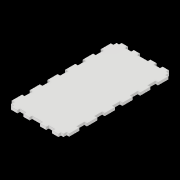
# Autodesk Inventor part: Bottom
Saved by Autodesk Inventor 2018 (Build 220112000, 112)
## iProperties
Created: 2018-03-12
Part Number: Bottom
Material: UHMW, White
Document SubType Name: Modeling
Designer: gaine
Density: 0.94 g/cm^3
Appearance: Smooth - White
Author: gaine
Autodesk Inventor part; units mm, degrees
ref_plane "YZ Plane" through (0, 0, 0) normal (1, 0, 0) x (0, 1, 0)
ref_plane "XZ Plane" through (0, 0, 0) normal (0, 1, 0) x (-1, 0, 0)
ref_plane "XY Plane" through (0, 0, 0) normal (0, 0, 1) x (1, 0, 0)
sketch "Sketch1" plane through (0, 0, 0) normal (0, 1, 0) x (-1, 0, 0)
  line L0 (36.5552, 136.6167) -> (36.5552, 130.2667)
  line L1 (21.3152, 130.2667) -> (21.3152, 136.6167)
  line L2 (58.1452, 96.9292) -> (64.4952, 96.9292)
  line L3 (64.4952, 77.8792) -> (58.1452, 77.8792)
  line L4 (58.1452, 52.4792) -> (64.4952, 52.4792)
  line L5 (64.4952, 33.4292) -> (58.1452, 33.4292)
  line L6 (58.1452, 8.0292) -> (64.4952, 8.0292)
  line L7 (64.4952, -1.4958) -> (-62.2762, -1.4958) construction
  line L8 (-7.1455, 136.6167) -> (-7.1455, -139.6083) construction
  line L9 (58.1452, 96.9292) -> (58.1452, 77.8792)
  line L10 (58.1452, 33.4292) -> (58.1452, 52.4792)
  line L11 (36.5552, 130.2667) -> (21.3152, 130.2667)
  line L12 (-50.8462, 136.6167) -> (-50.8462, 130.2667)
  line L13 (-20.3662, 136.6167) -> (-20.3662, 130.2667)
  line L14 (-35.6062, 130.2667) -> (-35.6062, 136.6167)
  line L15 (-78.7862, 122.3292) -> (-72.4362, 122.3292)
  line L16 (-72.4362, 96.9292) -> (-78.7862, 96.9292)
  line L17 (-78.7862, 77.8792) -> (-72.4362, 77.8792)
  line L18 (-72.4362, 52.4792) -> (-78.7862, 52.4792)
  line L19 (-78.7862, 33.4292) -> (-72.4362, 33.4292)
  line L20 (-72.4362, 8.0292) -> (-78.7862, 8.0292)
  line L21 (-72.4362, 96.9292) -> (-72.4362, 77.8792)
  line L22 (-72.4362, 33.4292) -> (-72.4362, 52.4792)
  line L23 (-50.8462, 130.2667) -> (-35.6062, 130.2667)
  line L24 (36.5552, -139.6083) -> (36.5552, -133.2583)
  line L25 (6.0752, -139.6083) -> (6.0752, -133.2583)
  line L26 (21.3152, -133.2583) -> (21.3152, -139.6083)
  line L27 (64.4952, -125.3208) -> (58.1452, -125.3208)
  line L28 (58.1452, -99.9208) -> (64.4952, -99.9208)
  line L29 (64.4952, -80.8708) -> (58.1452, -80.8708)
  line L30 (58.1452, -55.4708) -> (64.4952, -55.4708)
  line L31 (64.4952, -36.4208) -> (58.1452, -36.4208)
  line L32 (58.1452, -11.0208) -> (64.4952, -11.0208)
  line L33 (-7.1455, -139.6083) -> (-7.1455, 136.6167) construction
  line L34 (58.1452, -99.9208) -> (58.1452, -80.8708)
  line L35 (58.1452, -36.4208) -> (58.1452, -55.4708)
  line L36 (36.5552, -133.2583) -> (21.3152, -133.2583)
  line L37 (-72.4362, -55.4708) -> (-78.7862, -55.4708)
  line L38 (-78.7862, -80.8708) -> (-72.4362, -80.8708)
  line L39 (-72.4362, -99.9208) -> (-72.4362, -80.8708)
  line L40 (-50.8462, -139.6083) -> (-50.8462, -133.2583)
  line L41 (-20.3662, -139.6083) -> (-20.3662, -133.2583)
  line L42 (-35.6062, -133.2583) -> (-35.6062, -139.6083)
  line L43 (-72.4362, -99.9208) -> (-78.7862, -99.9208)
  line L44 (-78.7862, -125.3208) -> (-72.4362, -125.3208)
  line L45 (-50.8462, -133.2583) -> (-35.6062, -133.2583)
  line L46 (-72.4362, -36.4208) -> (-72.4362, -55.4708)
  line L47 (-78.7862, -36.4208) -> (-72.4362, -36.4208)
  line L48 (-72.4362, -11.0208) -> (-78.7862, -11.0208)
  line L49 (51.7952, 136.6167) -> (36.5552, 136.6167)
  line L50 (-20.3662, 136.6167) -> (-35.6062, 136.6167)
  line L51 (-50.8462, 136.6167) -> (-66.0862, 136.6167)
  line L52 (64.4952, 96.9292) -> (64.4952, 122.3292)
  line L53 (64.4952, 52.4792) -> (64.4952, 77.8792)
  line L54 (58.1452, 8.0292) -> (58.1452, -11.0208)
  line L55 (64.4952, 8.0292) -> (64.4952, 33.4292)
  line L56 (64.4952, -36.4208) -> (64.4952, -11.0208)
  line L57 (64.4952, -80.8708) -> (64.4952, -55.4708)
  line L58 (58.1452, -125.3208) -> (58.1452, -133.2583)
  line L59 (-72.4362, -133.2583) -> (-72.4362, -125.3208)
  line L60 (-72.4362, 8.0292) -> (-72.4362, -11.0208)
  line L61 (-72.4362, 122.3292) -> (-72.4362, 130.2667)
  line L62 (-78.7862, 122.3292) -> (-78.7862, 96.9292)
  line L63 (-78.7862, 77.8792) -> (-78.7862, 52.4792)
  line L64 (-78.7862, 33.4292) -> (-78.7862, 8.0292)
  line L65 (-78.7862, -11.0208) -> (-78.7862, -36.4208)
  line L66 (-78.7862, -55.4708) -> (-78.7862, -80.8708)
  line L67 (-78.7862, -99.9208) -> (-78.7862, -125.3208)
  line L68 (64.4952, -125.3208) -> (64.4952, -99.9208)
  line L69 (-66.0862, -139.6083) -> (-50.8462, -139.6083)
  line L70 (6.0752, -133.2583) -> (-20.3662, -133.2583)
  line L71 (-35.6062, -139.6083) -> (-20.3662, -139.6083)
  line L72 (6.0752, -139.6083) -> (21.3152, -139.6083)
  line L73 (36.5552, -139.6083) -> (51.7952, -139.6083)
  line L74 (58.1452, 130.2667) -> (51.7952, 130.2667)
  line L75 (51.7952, 130.2667) -> (51.7952, 136.6167)
  line L76 (-66.0862, 136.6167) -> (-66.0862, 130.2667)
  line L77 (-66.0862, -139.6083) -> (-66.0862, -133.2583)
  line L78 (51.7952, -139.6083) -> (51.7952, -133.2583)
  line L79 (6.0752, 130.2667) -> (-20.3662, 130.2667)
  line L80 (-66.0862, 130.2667) -> (-72.4362, 130.2667)
  line L81 (6.0752, 130.2667) -> (6.0752, 136.6167)
  line L82 (21.3152, 136.6167) -> (6.0752, 136.6167)
  line L83 (58.1452, 122.3292) -> (58.1452, 130.2667)
  line L84 (64.4952, 122.3292) -> (58.1452, 122.3292)
  line L85 (51.7952, -133.2583) -> (58.1452, -133.2583)
  line L86 (-66.0862, -133.2583) -> (-72.4362, -133.2583)
  point P0 (0, 0)
  point P1 (58.1452, 136.6167)
  dimension "d4" = 15.24
  dimension "d7" = 9.525
  dimension "d8" = 19.05
  dimension "d9" = 19.05
  dimension "d10" = 25.4
  dimension "d12" = 25.4
  dimension "d18" = 15.24
  dimension "d25" = 143.2814
  dimension "d27" = 6.35
  dimension "d28" = 15.24
  dimension "d29" = 6.35
  dimension "d30" = 15.24
  constraints: 174 end point, 59 symmetric about line, 50 parallel, 20 perpendicular, 11 horizontal, 9 collinear, 5 vertical, 1 point on line
  measures "d4" distance between parallel lines of L1 L0
  measures "d7" distance between parallel lines of L6 L7
  measures "d8" distance between parallel lines of L4 L5
  measures "d9" distance between parallel lines of L2 L3
  measures "d10" distance between parallel lines of L5 L6
  measures "d12" distance between parallel lines of L4 L3
  measures "d18" distance between parallel lines of L75 L0
  measures "d25" distance between parallel lines of L62 L52
  measures "d27" distance between parallel lines of L75 L83
  measures "d28" distance between parallel lines of L81 L1
  measures "d29" distance between parallel lines of L83 L52
  measures "d30" distance between parallel lines of L76 L12
extrude "Extrusion2" add sketch "Sketch1" along normal blind 6.35
equation "\"d4\" = d3"
equation "\"d8\" = 2 * d7"
equation "\"d9\" = d8"
equation "\"d10\" = d12"
equation "\"d12\" = d11"
equation "\"d30\" = d18"
equation "\"d3\" = 15.24"
equation "\"d11\" = 25.4"
body "Solid2"
